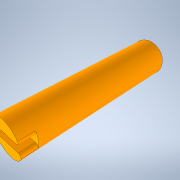
# Autodesk Inventor part: Шпунтик
Saved by Autodesk Inventor 2021.1 (Build 251245010, 245A)
## iProperties
Created: 2026-05-13
Part Number: Шпунтик
Material: Типовые
Document SubType Name: Modeling
Designer: Андрей Тарасов
Density: 1 g/cm^3
Appearance: По умолчанию
Author: Андрей Тарасов
Autodesk Inventor part; units mm, degrees
ref_plane "YZ Plane" through (0, 0, 0) normal (1, 0, 0) x (0, 1, 0)
ref_plane "XZ Plane" through (0, 0, 0) normal (0, 1, 0) x (-1, 0, 0)
ref_plane "XY Plane" through (0, 0, 0) normal (0, 0, 1) x (1, 0, 0)
sketch "Эскиз1" plane through (0, 0, 0) normal (0, 0, 1) x (1, 0, 0)
  circle A0 centre (0, 0) radius 2.55
  dimension "d0" = 5.1
  constraints: 1 centre point, 1 coincident
  measures "d0" diameter of A0
extrude "Выдавливание1" add sketch "Эскиз1" along normal blind 24
sketch "Эскиз2" plane through (0, 0, 24) normal (0, 0, 1) x (1, 0, 0)
  line L0 (2.55, -0.6) -> (-2.55, -0.6)
  line L1 (-2.55, -0.6) -> (-2.55, 0.6)
  line L2 (-2.55, 0.6) -> (2.55, 0.6)
  line L3 (2.55, 0.6) -> (2.55, -0.6)
  line L4 (2.55, -0.6) -> (-2.55, 0.6) construction
  line L5 (-2.55, -0.6) -> (2.55, 0.6) construction
  circle A0 centre (0, 0) radius 2.55 construction
  point P0 (0, 0)
  dimension "d3" = 1.2
  constraints: 12 end point, 3 midpoint, 2 parallel, 1 coincident, 1 horizontal, 1 perpendicular, 1 tangent
  measures "d3" distance of L2.end L0.start
extrude "Выдавливание2" cut sketch "Эскиз2" against normal blind 2
fillet "Сопряжение1" radius 0.4 4 edges at (2.4784, 0.6, 23) (-2.4784, 0.6, 23) (-2.4784, -0.6, 23) (2.4784, -0.6, 23)
